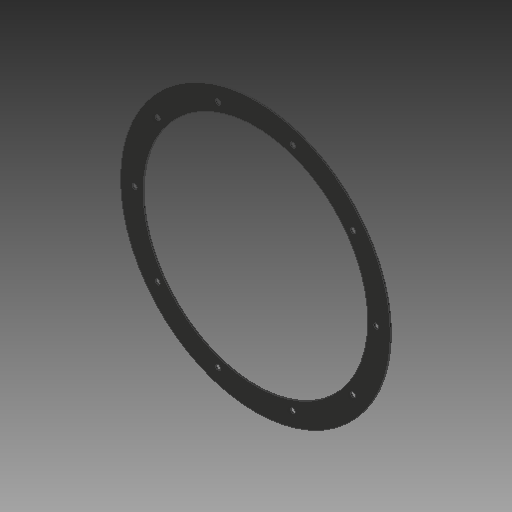
# Autodesk Inventor part: 1139_Outer Gasket_V1
Saved by Autodesk Inventor 2020 (Build 240168000, 168)
## iProperties
Created: 2019-05-13
Part Number: 1139_Outer Gasket_V1
Material: Rubber
Document SubType Name: Modeling
Designer: e22ma
Density: 0.93 g/cm^3
Appearance: Rubber - Black
Author: e22ma
Autodesk Inventor part; units mm, degrees
ref_plane "YZ Plane" through (0, 0, 0) normal (1, 0, 0) x (0, 1, 0)
ref_plane "XZ Plane" through (0, 0, 0) normal (0, 1, 0) x (-1, 0, 0)
ref_plane "Work Plane1" through (0, 0, 0) normal (0, 0, 1) x (1, 0, 0)
sketch "Sketch1" plane through (0, 0, 0) normal (0, 0, 1) x (1, 0, 0)
  circle A0 centre (26.4627, -50.6671) radius 1.8415 projected
  circle A1 centre (69.5627, -81.9811) radius 1.8415 projected
  circle A2 centre (122.8373, -81.9811) radius 1.8415 projected
  circle A3 centre (165.9373, -50.6671) radius 1.8415 projected
  circle A4 centre (182.4, 0) radius 1.8415 projected
  circle A5 centre (165.9373, 50.6671) radius 1.8415 projected
  circle A6 centre (122.8373, 81.9811) radius 1.8415 projected
  circle A7 centre (69.5627, 81.9811) radius 1.8415 projected
  circle A8 centre (26.4627, 50.6671) radius 1.8415 projected
  circle A9 centre (10, 0) radius 1.8415 projected
  circle A10 centre (96.2, 0) radius 80.1116 projected
  circle A11 centre (96.2, 0) radius 96.2 projected
  point P0 (0, 0)
  constraints: 1 horizontal alignment
extrude "Extrusion1" add sketch "Sketch1" along normal blind 0.7937
body "Solid1"
